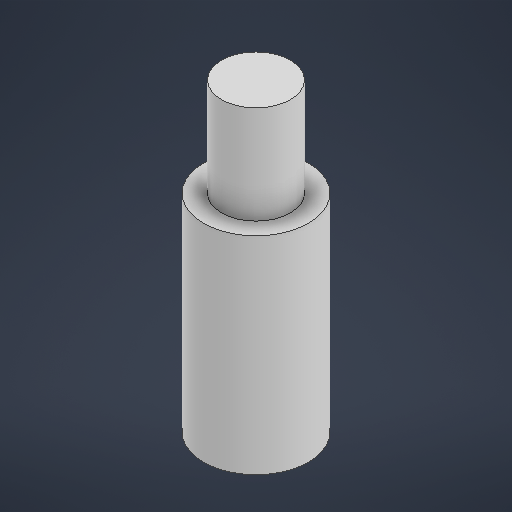
# Autodesk Inventor part: v3 adaptor
Saved by Autodesk Inventor 2026.2 (Build 302298000, 298)
## iProperties
Created: 2026-08-01
Part Number: v3 adaptor
Material: Generic
Document SubType Name: Modeling
Designer: Graeme
Density: 1 g/cm^3
Appearance: Default
Author: Graeme
## iProperties of the stored document v6 Knob extender long_3DPrint.ipt
Created: 2026-08-08
Part Number: v6 Knob extender long_3DPrint
Material: Generic
Document SubType Name: Modeling
Designer: Graeme
Density: 1 g/cm^3
Appearance: Default
Author: Graeme
Autodesk Inventor part; units mm, degrees
ref_plane "YZ Plane" through (0, 0, 0) normal (1, 0, 0) x (0, 1, 0)
ref_plane "XZ Plane" through (0, 0, 0) normal (0, 1, 0) x (-1, 0, 0)
ref_plane "XY Plane" through (0, 0, 0) normal (0, 0, 1) x (1, 0, 0)
sketch "Sketch1" plane through (0, 0, 0) normal (0, 1, 0) x (-1, 0, 0)
  point P0 (0, 0)
sketch "Sketch2" plane through (0, 0, 0) normal (0, 1, 0) x (-1, 0, 0)
  circle A0 centre (0, 0) radius 4.8
  dimension "d0" = 9.6
  constraints: 1 centre point, 1 coincident
  measures "d0" diameter of A0
extrude "Extrusion1" add sketch "Sketch2" along normal blind 19
sketch "Sketch3" plane through (0, 19, 0) normal (0, 1, 0) x (1, 0, 0)
  circle A0 centre (0, 0) radius 3
  line L0 (-2.6263, 1.45) -> (2.6263, 1.45)
  circle A1 centre (0, 0) radius 3.15
  point P0 (0, 1.45)
  dimension "d3" = 6
  dimension "d4" = 1.45
  dimension "d13" = 6.3
  constraints: 2 centre point, 2 coincident, 2 end point, 2 point on circle, 1 horizontal, 1 midpoint
  measures "d3" diameter of A0
  measures "d4" distance of point (0, 1.45) A0.centre
  measures "d13" diameter of A1
sketch "shaft cutout" plane through (0, 0, 0) normal (0, -1, 0) x (1, 0, 0)
  circle A0 centre (0, 0) radius 3.075
  line L0 (2.7117, -1.45) -> (-2.7117, -1.45)
  point P0 (0, -1.45)
  point P1 (0, -1.45)
  dimension "d7" = 6.15
  constraints: 2 coincident, 2 end point, 1 horizontal, 1 midpoint, 3 other
sketch "top spacer" plane through (0, 0, 0) normal (0, -1, 0) x (1, 0, 0)
  circle A0 centre (0, 0) radius 3.5
  dimension "d10" = 7
  constraints: 1 centre point, 1 coincident
  measures "d10" diameter of A0
extrude "Extrusion6" cut sketch "shaft cutout" against normal blind 9 contours A0 L0 picked at (0.9722, -0.3362)
extrude "Extrusion7" cut sketch "top spacer" against normal blind 3
extrude "Extrusion8" add sketch "Sketch3" along normal blind 9 contours A0 L0 | L0 A0 | A1
body "Solid1"
